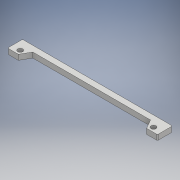
# Autodesk Inventor part: EsbarrosCarro
Saved by Autodesk Inventor 2018 (Build 220112000, 112)
## iProperties
Created: 2018-07-24
Part Number: EsbarrosCarro
Material: Genérico
Document SubType Name: Modeling
Designer: Usuario
Density: 1 g/cm^3
Appearance: Padrão
Mass: 59.3024 g
Surface Area: 209.133 cm^2
Volume: 59.3024 cm^3
Author: Usuario
Autodesk Inventor part; units mm, degrees
ref_plane "YZ Plane" through (0, 0, 0) normal (1, 0, 0) x (0, 1, 0)
ref_plane "XZ Plane" through (0, 0, 0) normal (0, 1, 0) x (-1, 0, 0)
ref_plane "XY Plane" through (0, 0, 0) normal (0, 0, 1) x (1, 0, 0)
sketch "Esboço1" plane through (0, 0, 0) normal (0, 0, 1) x (1, 0, 0)
  line L0 (-18, 25.5) -> (338, 25.5)
  line L1 (340, 23.5) -> (340, -8.5)
  line L2 (-20, -8.5) -> (-20, 23.5)
  circle A0 centre (0, 0) radius 5.995 construction
  circle A1 centre (320, 0) radius 5.995 construction
  line L3 (6, -10.5) -> (18.7017, 11.5)
  line L4 (6, -10.5) -> (31.4034, -10.5) construction
  line L5 (18.7017, 11.5) -> (161.7689, 11.5)
  line L6 (160, 31.3493) -> (160, -25.519) construction
  line L7 (314, -10.5) -> (301.2983, 11.5)
  line L8 (301.2983, 11.5) -> (161.7689, 11.5)
  line L9 (-18, 25.5) -> (-20, 23.5)
  line L10 (-20, -8.5) -> (-18, -10.5)
  line L11 (338, 25.5) -> (340, 23.5)
  line L12 (338, -10.5) -> (340, -8.5)
  line L13 (338, -10.5) -> (314, -10.5)
  line L14 (6, -10.5) -> (-18, -10.5)
  circle A2 centre (0, 0) radius 6
  circle A3 centre (320, 0) radius 6
  point P0 (340, -10.5)
  point P1 (340, 25.5)
  point P2 (-20, -10.5)
  point P3 (-20, 25.5)
  dimension "d0" = 36
  dimension "d2" = 2
  dimension "d3" = 2
  dimension "d4" = 2
  dimension "d5" = 2
  dimension "d6" = 2
  dimension "d7" = 2
  dimension "d8" = 2
  dimension "d9" = 2
  dimension "d10" = 12
  dimension "d11" = 12
  dimension "d14" = 120
  dimension "d15" = 14
  dimension "d16" = 24
  constraints: 30 end point, 6 point on line, 4 horizontal, 4 parallel, 3 vertical, 2 centre point, 2 coincident, 2 symmetric about line, 1 equal length, 1 perpendicular
  measures "d0" distance of point (340, 25.5) point (340, -10.5)
  measures "d2" distance of L0.start point (-20, 25.5)
  measures "d3" distance of L2.end point (-20, 25.5)
  measures "d4" distance of L2.start point (-20, -10.5)
  measures "d5" distance of L10.end point (-20, -10.5)
  measures "d6" distance of L0.end point (340, 25.5)
  measures "d7" distance of L1.start point (340, 25.5)
  measures "d8" distance of L12.start point (340, -10.5)
  measures "d9" distance of L1.end point (340, -10.5)
  measures "d10" diameter of A2
  measures "d11" diameter of A3
  measures "d14" angle of L14 L3
  measures "d15" distance between parallel lines of L8 L0
  measures "d16" distance of L3.start L10.end
extrude "Extrusão1" add sketch "Esboço1" against normal blind 12.52
equation "\"d3\" = d2"
equation "\"d4\" = d2"
equation "\"d5\" = d4"
equation "\"d6\" = d2"
equation "\"d7\" = d6"
equation "\"d8\" = d2"
equation "\"d9\" = d8"
